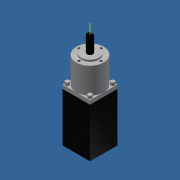
# Autodesk Inventor part: Nema17 Geared
Saved by Autodesk Inventor 2014 SP2 (Build 180246200, 246)
## iProperties
Created: 2014-12-12
Part Number: Nema17 Geared
Material: Stahl
Document SubType Name: Modeling
Designer: 4ndreas
Density: 7.85 g/cm^3
Appearance: Stahl
Mass: 466.362 g
Surface Area: 122.914 cm^2
Volume: 59.4092 cm^3
Author: 4ndreas
Autodesk Inventor part; units mm, degrees
ref_plane "YZ Plane" through (0, 0, 0) normal (1, 0, 0) x (0, 1, 0)
ref_plane "XZ Plane" through (0, 0, 0) normal (0, 1, 0) x (-1, 0, 0)
ref_plane "XY Plane" through (0, 0, 0) normal (0, 0, 1) x (1, 0, 0)
sketch "Skizze1" plane through (0, 0, 0) normal (0, 0, 1) x (1, 0, 0)
  circle A0 centre (0, 0) radius 14
  dimension "d0" = 28
  constraints: 1 centre point, 1 coincident
  measures "d0" diameter of A0
extrude "Extrusion1" add sketch "Skizze1" along normal blind 26.35
sketch "Skizze2" plane through (0, 0, 26.35) normal (0, 0, 1) x (1, 0, 0)
  circle A0 centre (0, 0) radius 14 projected
  circle A1 centre (0, 0) radius 9
  dimension "d3" = 18
  constraints: 1 centre point, 1 coincident
  measures "d3" diameter of A1
extrude "Extrusion2" add sketch "Skizze2" along normal blind 1.75 contours A1
sketch "Skizze3" plane through (0, 0, 26.35) normal (0, 0, 1) x (1, 0, 0)
  circle A0 centre (0, 0) radius 14 projected
  line L0 (0, 0) -> (-11.25, 0) construction
  dimension "d6" = 11.25
  constraints: 2 end point, 1 horizontal
  measures "d6" distance of L0.start L0.end
hole "Bohrung1" at (-11.25, 0, 26.35) direction (0, 0, -1) diameter 2.459 depth 8 tip angle 118 thread size "M3x0.5" class "6H" standard "ANSI Metric M Profile"
sketch "Skizze4" plane through (0, 0, 28.1) normal (0, 0, 1) x (1, 0, 0)
  circle A0 centre (0, 0) radius 9 projected
  circle A1 centre (0, 0) radius 3
  dimension "d14" = 6
  constraints: 1 centre point, 1 coincident
  measures "d14" diameter of A1
extrude "Extrusion3" add sketch "Skizze4" along normal blind 16 contours A1
sketch "Skizze5" plane through (0, 0, 44.1) normal (0, 0, 1) x (1, 0, 0)
  circle A0 centre (0, 0) radius 3 projected
  line L0 (-2.2361, 2) -> (2.2361, 2)
  dimension "d17" = 5
  constraints: 2 end point, 2 point on circle, 1 horizontal
extrude "Extrusion4" cut sketch "Skizze5" against normal blind 12.5 contours L0 A0 picked at (-0.5653, 2.1582)
pattern_circular "Runde Anordnung1" count 4 over 360 about axis through (0, 0, 28.1) along (0, 0, 1) of "Bohrung1"
sketch "Skizze6" plane through (0, 0, 0) normal (0, 0, -1) x (-1, 0, 0)
  circle A0 centre (0, 0) radius 14 projected
  line L0 (-14, 14) -> (14, 14)
  line L1 (14, 14) -> (14, -14)
  line L2 (14, -14) -> (-14, -14)
  line L3 (-14, -14) -> (-14, 14)
  constraints: 8 end point, 4 tangent, 2 parallel, 1 horizontal, 1 perpendicular
extrude "Extrusion5" add sketch "Skizze6" along normal blind 4
sketch "Skizze7" plane through (0, 0, 0) normal (0, 0, 1) x (1, 0, 0)
  line L0 (0, 14) -> (-14, 14) projected
  line L1 (-14, 14) -> (-14, 0) projected
  circle A0 centre (-11.598, 11.598) radius 2.402
  circle A1 centre (0, 0) radius 14 projected
  circle A2 centre (-11.598, 11.598) radius 2
  dimension "d25" = 4
  constraints: 3 tangent, 2 centre point, 1 coincident
  measures "d25" diameter of A2
extrude "Extrusion6" add sketch "Skizze7" along normal blind 2.9 contours A2
pattern_circular "Runde Anordnung3" count 4 over 360 about axis through (0, 0, 0) along (0, 0, 1) of "Extrusion6"
sketch "Skizze8" plane through (0, 0, -4) normal (0, 0, -1) x (-1, 0, 0)
  line L0 (14, 14) -> (-14, 14) projected
  line L1 (-14, 14) -> (-14, -14) projected
  line L2 (-14, -14) -> (14, -14) projected
  line L3 (14, -14) -> (14, 14) projected
  point P0 (0, 0)
extrude "Extrusion7" add sketch "Skizze8" along normal blind 50 separate body
